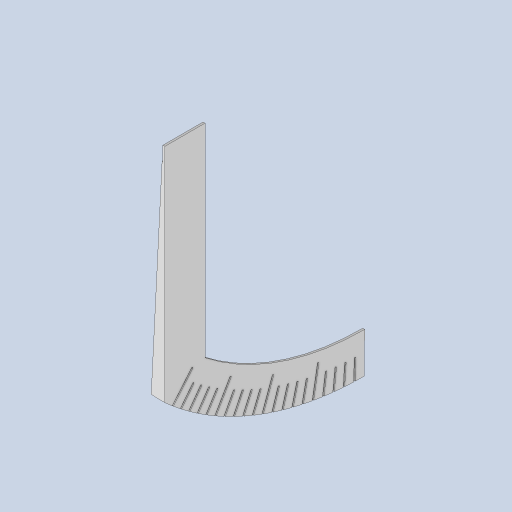
# Autodesk Inventor part: elev_angler
Saved by Autodesk Inventor 2024.1 (Build 281209000, 209)
## iProperties
Created: 2023-12-04
Part Number: elev_angler
Material: Generic
Document SubType Name: Modeling
Designer: dsdan
Density: 1 g/cm^3
Appearance: Default
Author: dsdan
Autodesk Inventor part; units mm, degrees
ref_plane "YZ Plane" through (0, 0, 0) normal (1, 0, 0) x (0, 1, 0)
ref_plane "XZ Plane" through (0, 0, 0) normal (0, 1, 0) x (-1, 0, 0)
ref_plane "XY Plane" through (0, 0, 0) normal (0, 0, 1) x (1, 0, 0)
sketch "Sketch1" plane through (0, 0, 0) normal (1, 0, 0) x (0, 1, 0)
  circle A0 centre (0, 0) radius 148.5
  line L0 (110.3263, 99.4) -> (-110.3263, 99.4)
  line L1 (0, 99.4) -> (0, 79.4)
  line L2 (0, 79.4) -> (-101.0341, 79.4)
  circle A1 centre (0, 0) radius 128.5
  line L3 (0, -148.5) -> (0, -128.5)
  point P0 (0, 99.4)
  dimension "d0" = 297
  dimension "d1" = 99.4
  dimension "d2" = 20
  dimension "d3" = 20
  dimension "d4" = 0
  constraints: 8 end point, 5 point on circle, 2 centre point, 2 midpoint, 2 vertical, 1 coincident, 1 horizontal, 1 perpendicular, 1 point on line
  measures "d0" diameter of A0
  measures "d1" distance from line of A0.centre L0
  measures "d2" radial gap between concentric circles of A0 A1
  measures "d3" distance between parallel lines of L0 L2
  measures "d4" distance from line of point (0, 99.4) L1
extrude "Extrusion1" add sketch "Sketch1" along normal mid plane 1 contours A0 L0 A1 L3 | L0 L1 L2 A1 picked at (-141.6144, 0.3829) picked at (-27.1455, 92.7333)
sketch "Sketch2" plane through (0.5, 0, 0) normal (1, 0, 0) x (0, 0, -1)
  line L0 (138.4156, -4.8336) -> (148.4095, -5.1826) construction
  line L1 (138.4287, -4.4588) -> (148.4226, -4.8078)
  line L2 (148.3965, -5.5573) -> (138.4025, -5.2084)
  arc A0 (138.4287, -4.4588) -> (138.4025, -5.2084) centre (138.4156, -4.8336) ccw
  arc A1 (148.3965, -5.5573) -> (148.4226, -4.8078) centre (148.4095, -5.1826) ccw
  arc A2 (-99.4, -110.3263) -> (148.5, 0) centre (0, 0) ccw projected
  line L3 (148.5, 0) -> (128.5, 0) projected
  line L4 (146.244, -25.7868) -> (131.4718, -23.182) construction
  line L5 (146.3091, -25.4175) -> (131.537, -22.8127)
  line L6 (131.4067, -23.5513) -> (146.1788, -26.1561)
  arc A3 (146.1788, -26.1561) -> (146.3091, -25.4175) centre (146.244, -25.7868) ccw
  arc A4 (131.537, -22.8127) -> (131.4067, -23.5513) centre (131.4718, -23.182) ccw
  point P0 (143.4126, -5.0081)
  point P1 (148.396, -5.5573)
  point P2 (148.4222, -4.8078)
  point P3 (138.8579, -24.4844)
  point P4 (146.1784, -26.156)
  point P5 (146.3086, -25.4174)
  dimension "d7" = 10
  dimension "d8" = 0.75
  dimension "d9" = 2
  dimension "d15" = 0.75
  dimension "d16" = 10
  dimension "d17" = 15
  constraints: 16 end point, 10 point on circle, 8 tangent, 4 centre point, 2 midpoint, 2 parallel, 2 point on line
  measures "d7" distance of L0.start L0.end
  measures "d8" distance between parallel lines of L2 L1
  measures "d9" angle of L3 L0
  measures "d15" diameter of A4
  measures "d16" angle of L3 L4
  measures "d17" distance of L4.start L4.end
extrude "Extrusion2" cut sketch "Sketch2" against normal blind 0.45 contours L1 A2 L2 A0
extrude "Extrusion3" cut sketch "Sketch2" against normal blind 0.45 contours L6 A4 L5 A2
pattern_circular "Circular Pattern1" count 65 over 128 about axis through (-10, 0, 0) along (-1, 0, 0) of "Extrusion2"
pattern_circular "Circular Pattern2" count 13 over 120 about axis through (-10, 0, 0) along (-1, 0, 0) of "Extrusion3"
sketch "Sketch3" plane through (-0.5, 0, 0) normal (-1, 0, 0) x (0, 0, 1)
  arc A0 (-148.5, 0) -> (99.4, -110.3263) centre (0, 0) ccw projected
  arc A1 (-146.7, 0) -> (112.3263, -94.3594) centre (0, 0) ccw
  line L0 (-148.5, 0) -> (-128.5, 0) projected
  line L1 (99.4, -110.3263) -> (99.4, 0) projected
  line L2 (-243.6606, 0) -> (171.6574, 0) projected
  point P0 (99.4, -107.8913)
  dimension "d23" = 1.8
  constraints: 2 point on circle, 1 centre point
  measures "d23" radial gap between concentric circles of A0 A1
revolve "Revolution1" add sketch "Sketch3" angle 3 about axis through (-0.5, 0, -10) along (0, 0, -1) contours L0 A1 L1 A0
sketch "Sketch4" plane through (0.5, -110.3263, 99.4) normal (0, 0, 1) x (1, 0, 0)
  circle A0 centre (-0.5, 110.3263) radius 2.95
  line L0 (-1, 0) -> (0, 0) projected
  line L1 (0, 110.3263) -> (0, 0) projected
  line L2 (-1, 110.3263) -> (0, 110.3263) projected
  line L3 (-1, 2.435) -> (-1, 110.3263) projected
  line L4 (0.075, -0.075) -> (-1, -0.075)
  arc A1 (-6.9581, 0.083) -> (-1, -0.075) centre (-1, 112.3372) ccw
  line L5 (-6.9581, 0.083) -> (-6.8239, 2.6445)
  arc A2 (-6.8239, 2.6445) -> (-1.075, 2.49) centre (-1, 112.3372) ccw
  line L6 (-1.075, 2.49) -> (-1.075, 110.2513)
  line L7 (-1.075, 110.2513) -> (0.075, 110.2513)
  line L8 (0.075, 110.2513) -> (0.075, -0.075)
  arc A3 (-6.6466, 2.5829) -> (-1, 2.435) centre (-1, 110.3263) ccw projected
  line L9 (-6.774, 0.1512) -> (-6.6466, 2.5829) projected
  arc A4 (-6.774, 0.1512) -> (-1, 0) centre (-1, 110.3263) ccw projected
  point P0 (0.075, 107.4329)
  point P1 (-1.075, 107.4329)
  dimension "d25" = 5.9
  dimension "d26" = 0.075
  constraints: 10 end point, 4 point on circle, 3 centre point, 1 midpoint, 2 other
  measures "d25" diameter of A0
  measures "d26" distance between parallel lines of L1 L8
extrude "Extrusion4" add sketch "Sketch4" along normal blind 5 and the other way blind 20 separate body contours A0 L8 L7 L1 L2 L3 L6 | L3 L2 L1 L7
split body "Split2" result two bodies by plane through (0, 0, 0) normal (0, 0, 1) bodies 1 first body at (0, -33.678, 86.0667)
ref_plane "Work Plane4" through (0, 0, -128.5) normal (0, 0, -1) x (-1, 0, 0)
sketch "Sketch6" plane through (0, 0, -128.5) normal (0, 0, 1) x (1, 0, 0)
  line L0 (0.05, -148.5) -> (-0.5, -148.5) projected
  line L1 (-0.5, 0) -> (-0.5, -148.5) projected
  line L2 (-0.5, 0) -> (0.5, 0) projected
  line L3 (0.5, -4.8078) -> (0.5, 0) projected
  line L4 (0.5, -4.8078) -> (0.05, -4.8078) projected
  line L5 (0.05, -4.8078) -> (0.05, -5.5573) projected
  line L6 (0.05, -5.5573) -> (0.5, -5.5573) projected
  line L7 (0.5, -9.9847) -> (0.5, -5.5573) projected
  line L8 (0.5, -9.9847) -> (0.05, -9.9847) projected
  line L9 (0.05, -9.9847) -> (0.05, -10.7329) projected
  line L10 (0.05, -10.7329) -> (0.5, -10.7329) projected
  line L11 (0.5, -15.1495) -> (0.5, -10.7329) projected
  line L12 (0.5, -15.1495) -> (0.05, -15.1495) projected
  line L13 (0.05, -15.1495) -> (0.05, -15.8954) projected
  line L14 (0.05, -15.8954) -> (0.5, -15.8954) projected
  line L15 (0.5, -20.2958) -> (0.5, -15.8954) projected
  line L16 (0.5, -20.2958) -> (0.05, -20.2958) projected
  line L17 (0.05, -20.2958) -> (0.05, -21.0385) projected
  line L18 (0.05, -21.0385) -> (0.5, -21.0385) projected
  line L19 (0.5, -25.4174) -> (0.5, -21.0385) projected
  line L20 (0.5, -25.4174) -> (0.05, -25.4174) projected
  line L21 (0.05, -25.4174) -> (0.05, -26.156) projected
  line L22 (0.05, -26.156) -> (0.5, -26.156) projected
  line L23 (0.5, -30.508) -> (0.5, -26.156) projected
  line L24 (0.5, -30.508) -> (0.05, -30.508) projected
  line L25 (0.05, -30.508) -> (0.05, -31.2416) projected
  line L26 (0.05, -31.2416) -> (0.5, -31.2416) projected
  line L27 (0.5, -35.5614) -> (0.5, -31.2416) projected
  line L28 (0.5, -35.5614) -> (0.05, -35.5614) projected
  line L29 (0.05, -35.5614) -> (0.05, -36.2891) projected
  line L30 (0.05, -36.2891) -> (0.5, -36.2891) projected
  line L31 (0.5, -40.5715) -> (0.5, -36.2891) projected
  line L32 (0.5, -40.5715) -> (0.05, -40.5715) projected
  line L33 (0.05, -40.5715) -> (0.05, -41.2925) projected
  line L34 (0.05, -41.2925) -> (0.5, -41.2925) projected
  line L35 (0.5, -45.5322) -> (0.5, -41.2925) projected
  line L36 (0.5, -45.5322) -> (0.05, -45.5322) projected
  line L37 (0.05, -45.5322) -> (0.05, -46.2455) projected
  line L38 (0.05, -46.2455) -> (0.5, -46.2455) projected
  line L39 (0.5, -50.4374) -> (0.5, -46.2455) projected
  line L40 (0.5, -50.4374) -> (0.05, -50.4374) projected
  line L41 (0.05, -50.4374) -> (0.05, -51.1422) projected
  line L42 (0.05, -51.1422) -> (0.5, -51.1422) projected
  line L43 (0.5, -55.2812) -> (0.5, -51.1422) projected
  line L44 (0.5, -55.2812) -> (0.05, -55.2812) projected
  line L45 (0.05, -55.2812) -> (0.05, -55.9766) projected
  line L46 (0.05, -55.9766) -> (0.5, -55.9766) projected
  line L47 (0.5, -60.0576) -> (0.5, -55.9766) projected
  line L48 (0.5, -60.0576) -> (0.05, -60.0576) projected
  line L49 (0.05, -60.0576) -> (0.05, -60.7428) projected
  line L50 (0.05, -60.7428) -> (0.5, -60.7428) projected
  line L51 (0.5, -64.7609) -> (0.5, -60.7428) projected
  line L52 (0.5, -64.7609) -> (0.05, -64.7609) projected
  line L53 (0.05, -64.7609) -> (0.05, -65.435) projected
  line L54 (0.05, -65.435) -> (0.5, -65.435) projected
  line L55 (0.5, -69.3852) -> (0.5, -65.435) projected
  line L56 (0.5, -69.3852) -> (0.05, -69.3852) projected
  line L57 (0.05, -69.3852) -> (0.05, -70.0474) projected
  line L58 (0.05, -70.0474) -> (0.5, -70.0474) projected
  line L59 (0.5, -73.925) -> (0.5, -70.0474) projected
  line L60 (0.5, -73.925) -> (0.05, -73.925) projected
  line L61 (0.05, -73.925) -> (0.05, -74.5745) projected
  line L62 (0.05, -74.5745) -> (0.5, -74.5745) projected
  line L63 (0.5, -78.3747) -> (0.5, -74.5745) projected
  line L64 (0.5, -78.3747) -> (0.05, -78.3747) projected
  line L65 (0.05, -78.3747) -> (0.05, -79.0108) projected
  line L66 (0.05, -79.0108) -> (0.5, -79.0108) projected
  line L67 (0.5, -82.729) -> (0.5, -79.0108) projected
  line L68 (0.5, -82.729) -> (0.05, -82.729) projected
  line L69 (0.05, -82.729) -> (0.05, -83.3508) projected
  line L70 (0.05, -83.3508) -> (0.5, -83.3508) projected
  line L71 (0.5, -86.9825) -> (0.5, -83.3508) projected
  line L72 (0.5, -86.9825) -> (0.05, -86.9825) projected
  line L73 (0.05, -86.9825) -> (0.05, -87.5892) projected
  line L74 (0.05, -87.5892) -> (0.5, -87.5892) projected
  line L75 (0.5, -91.1299) -> (0.5, -87.5892) projected
  line L76 (0.5, -91.1299) -> (0.05, -91.1299) projected
  line L77 (0.05, -91.1299) -> (0.05, -91.7209) projected
  line L78 (0.05, -91.7209) -> (0.5, -91.7209) projected
  line L79 (0.5, -95.1664) -> (0.5, -91.7209) projected
  line L80 (0.5, -95.1664) -> (0.05, -95.1664) projected
  line L81 (0.05, -95.1664) -> (0.05, -95.7409) projected
  line L82 (0.05, -95.7409) -> (0.5, -95.7409) projected
  line L83 (0.5, -99.0869) -> (0.5, -95.7409) projected
  line L84 (0.5, -99.0869) -> (0.05, -99.0869) projected
  line L85 (0.05, -99.0869) -> (0.05, -99.6443) projected
  line L86 (0.05, -99.6443) -> (0.5, -99.6443) projected
  line L87 (0.5, -102.8867) -> (0.5, -99.6443) projected
  line L88 (0.5, -102.8867) -> (0.05, -102.8867) projected
  line L89 (0.05, -102.8867) -> (0.05, -103.4262) projected
  line L90 (0.05, -103.4262) -> (0.5, -103.4262) projected
  line L91 (0.5, -106.5611) -> (0.5, -103.4262) projected
  line L92 (0.5, -106.5611) -> (0.05, -106.5611) projected
  line L93 (0.05, -106.5611) -> (0.05, -107.0821) projected
  line L94 (0.05, -107.0821) -> (0.5, -107.0821) projected
  line L95 (0.5, -110.1057) -> (0.5, -107.0821) projected
  line L96 (0.5, -110.1057) -> (0.05, -110.1057) projected
  line L97 (0.05, -110.1057) -> (0.05, -110.6076) projected
  line L98 (0.05, -110.6076) -> (0.5, -110.6076) projected
  line L99 (0.5, -113.5162) -> (0.5, -110.6076) projected
  line L100 (0.5, -113.5162) -> (0.05, -113.5162) projected
  line L101 (0.05, -113.5162) -> (0.05, -113.9983) projected
  line L102 (0.05, -113.9983) -> (0.5, -113.9983) projected
  line L103 (0.5, -116.7884) -> (0.5, -113.9983) projected
  line L104 (0.5, -116.7884) -> (0.05, -116.7884) projected
  line L105 (0.05, -116.7884) -> (0.05, -117.2501) projected
  line L106 (0.05, -117.2501) -> (0.5, -117.2501) projected
  line L107 (0.5, -119.9182) -> (0.5, -117.2501) projected
  line L108 (0.5, -119.9182) -> (0.05, -119.9182) projected
  line L109 (0.05, -119.9182) -> (0.05, -120.3591) projected
  line L110 (0.05, -120.3591) -> (0.5, -120.3591) projected
  line L111 (0.5, -122.902) -> (0.5, -120.3591) projected
  line L112 (0.5, -122.902) -> (0.05, -122.902) projected
  line L113 (0.05, -122.902) -> (0.05, -123.3214) projected
  line L114 (0.05, -123.3214) -> (0.5, -123.3214) projected
  line L115 (0.5, -125.736) -> (0.5, -123.3214) projected
  line L116 (0.5, -125.736) -> (0.05, -125.736) projected
  line L117 (0.05, -125.736) -> (0.05, -126.1335) projected
  line L118 (0.05, -126.1335) -> (0.5, -126.1335) projected
  line L119 (0.5, -128.4169) -> (0.5, -126.1335) projected
  line L120 (0.5, -128.4169) -> (0.05, -128.4169) projected
  line L121 (0.05, -128.4169) -> (0.05, -128.7919) projected
  line L122 (0.05, -128.7919) -> (0.5, -128.7919) projected
  line L123 (0.5, -130.9412) -> (0.5, -128.7919) projected
  line L124 (0.5, -130.9412) -> (0.05, -130.9412) projected
  line L125 (0.05, -130.9412) -> (0.05, -131.2934) projected
  line L126 (0.05, -131.2934) -> (0.5, -131.2934) projected
  line L127 (0.5, -133.3061) -> (0.5, -131.2934) projected
  line L128 (0.5, -133.3061) -> (0.05, -133.3061) projected
  line L129 (0.05, -133.3061) -> (0.05, -133.6349) projected
  line L130 (0.05, -133.6349) -> (0.5, -133.6349) projected
  line L131 (0.5, -135.5085) -> (0.5, -133.6349) projected
  line L132 (0.5, -135.5085) -> (0.05, -135.5085) projected
  line L133 (0.05, -135.5085) -> (0.05, -135.8136) projected
  line L134 (0.05, -135.8136) -> (0.5, -135.8136) projected
  line L135 (0.5, -137.5459) -> (0.5, -135.8136) projected
  line L136 (0.5, -137.5459) -> (0.05, -137.5459) projected
  line L137 (0.05, -137.5459) -> (0.05, -137.8268) projected
  line L138 (0.05, -137.8268) -> (0.5, -137.8268) projected
  line L139 (0.5, -139.4157) -> (0.5, -137.8268) projected
  line L140 (0.5, -139.4157) -> (0.05, -139.4157) projected
  line L141 (0.05, -139.4157) -> (0.05, -139.6722) projected
  line L142 (0.05, -139.6722) -> (0.5, -139.6722) projected
  line L143 (0.5, -141.1156) -> (0.5, -139.6722) projected
  line L144 (0.5, -141.1156) -> (0.05, -141.1156) projected
  line L145 (0.05, -141.1156) -> (0.05, -141.3473) projected
  line L146 (0.05, -141.3473) -> (0.5, -141.3473) projected
  line L147 (0.5, -142.6435) -> (0.5, -141.3473) projected
  line L148 (0.5, -142.6435) -> (0.05, -142.6435) projected
  line L149 (0.05, -142.6435) -> (0.05, -142.8503) projected
  line L150 (0.05, -142.8503) -> (0.5, -142.8503) projected
  line L151 (0.5, -143.9977) -> (0.5, -142.8503) projected
  line L152 (0.5, -143.9977) -> (0.05, -143.9977) projected
  line L153 (0.05, -143.9977) -> (0.05, -144.1792) projected
  line L154 (0.05, -144.1792) -> (0.5, -144.1792) projected
  line L155 (0.5, -145.1765) -> (0.5, -144.1792) projected
  line L156 (0.5, -145.1765) -> (0.05, -145.1765) projected
  line L157 (0.05, -145.1765) -> (0.05, -145.3324) projected
  line L158 (0.05, -145.3324) -> (0.5, -145.3324) projected
  line L159 (0.5, -146.1784) -> (0.5, -145.3324) projected
  line L160 (0.5, -146.1784) -> (0.05, -146.1784) projected
  line L161 (0.05, -146.1784) -> (0.05, -146.3086) projected
  line L162 (0.05, -146.3086) -> (0.5, -146.3086) projected
  line L163 (0.5, -147.0021) -> (0.5, -146.3086) projected
  line L164 (0.5, -147.0021) -> (0.05, -147.0021) projected
  line L165 (0.05, -147.0021) -> (0.05, -147.1065) projected
  line L166 (0.05, -147.1065) -> (0.5, -147.1065) projected
  line L167 (0.5, -147.6468) -> (0.5, -147.1065) projected
  line L168 (0.5, -147.6468) -> (0.05, -147.6468) projected
  line L169 (0.05, -147.6468) -> (0.05, -147.7252) projected
  line L170 (0.05, -147.7252) -> (0.5, -147.7252) projected
  line L171 (0.5, -148.1116) -> (0.5, -147.7252) projected
  line L172 (0.5, -148.1116) -> (0.05, -148.1116) projected
  line L173 (0.05, -148.1116) -> (0.05, -148.1639) projected
  line L174 (0.05, -148.1639) -> (0.5, -148.1639) projected
  line L175 (0.5, -148.396) -> (0.5, -148.1639) projected
  line L176 (0.5, -148.396) -> (0.05, -148.396) projected
  line L177 (0.05, -148.396) -> (0.05, -148.4222) projected
  line L178 (0.05, -148.4222) -> (0.5, -148.4222) projected
  line L179 (0.5, -148.4995) -> (0.5, -148.4222) projected
  line L180 (0.5, -148.4995) -> (0.05, -148.4995) projected
  line L181 (0.05, -148.4995) -> (0.05, -148.5) projected
  circle A0 centre (0, 0) radius 3.5
  circle A1 centre (0, 0) radius 0.6
  line L182 (0, 0) -> (0, 0.5)
  line L183 (0, 0.5) -> (3.4641, 0.5)
  line L184 (0, 0.5) -> (-3.4641, 0.5)
  point P0 (0, 0.25)
  point P1 (-0.3317, 0.5)
  point P2 (0.3317, 0.5)
  dimension "d33" = 7
  dimension "d34" = 1.2
  dimension "d35" = 0.5
  dimension "d36" = 1
  constraints: 6 end point, 2 centre point, 2 coincident, 2 horizontal, 2 point on circle, 1 midpoint, 1 vertical
  measures "d33" diameter of A0
  measures "d34" diameter of A1
  measures "d35" distance of L182.start L182.end
  measures "d36" distance of L1.start L2.end
extrude "Extrusion5" add sketch "Sketch6" against normal blind 15 separate body contours A0 L183 A1 L184
sketch "Sketch7" plane through (0, 0, -143.5) normal (0, 0, -1) x (-1, 0, 0)
  arc A0 (3.4641, 0.5) -> (-3.4641, 0.5) centre (0, 0) ccw projected
  line L0 (-3.4641, 0.5) -> (3.4641, 0.5)
  line L1 (3.4641, 0.5) -> (3.4641, 6)
  line L2 (3.4641, 6) -> (-3.4641, 6)
  line L3 (-3.4641, 6) -> (-3.4641, 0.5)
  arc A1 (0.3317, 0.5) -> (-0.3317, 0.5) centre (0, 0) ccw projected
  line L4 (-4.5714, 3.05) -> (7.081, 3.05)
  line L5 (0.5, 0) -> (-0.5, 0) projected
  point P0 (0, 0)
  point P1 (-3.4641, 3.05)
  point P2 (3.4641, 3.05)
  dimension "d40" = 5.5
  dimension "d41" = 3.05
  constraints: 10 end point, 2 horizontal, 2 parallel, 1 perpendicular, 1 point on line
  measures "d40" distance between parallel lines of L0 L2
  measures "d41" distance between parallel lines of L5 L4
extrude "Extrusion6" add sketch "Sketch7" along normal blind 20 contours L4 A0 | A0 L4 L3 L2 L1 bodies 5
extrude "Extrusion7" add sketch "Sketch7" against normal up to surface (15 mm away) contours A0 L4 L1 | A0 L4 L3 L2 L1 | A0 L3 L4 bodies 5
sketch "Sketch8" plane through (-3.4641, 6, -143.5) normal (0, 1, 0) x (1, 0, 0)
  line L0 (3.4641, 16.0677) -> (3.4641, 9.0677) construction
  line L1 (1.4141, 16.0677) -> (1.4141, 9.0677)
  line L2 (5.5141, 9.0677) -> (5.5141, 16.0677)
  arc A0 (5.5141, 16.0677) -> (1.4141, 16.0677) centre (3.4641, 16.0677) ccw
  arc A1 (1.4141, 9.0677) -> (5.5141, 9.0677) centre (3.4641, 9.0677) ccw
  line L3 (0, 20) -> (6.9282, 20) projected
  point P0 (3.4641, -143.5)
  point P1 (3.4641, 12.5677)
  point P2 (3.4641, 20)
  point P3 (3.4641, 20)
  dimension "d46" = 4.1
  dimension "d47" = 7
  constraints: 8 end point, 4 point on circle, 4 tangent, 3 midpoint, 2 centre point, 1 parallel, 1 point on line, 1 vertical
  measures "d46" diameter of A1
  measures "d47" distance of L0.start L0.end
extrude "Extrusion8" cut sketch "Sketch8" against normal through all bodies 5
sketch "Sketch10" plane through (0.5, -110.3263, 99.4) normal (0, 0, 1) x (1, 0, 0)
  line L0 (-1, 2.435) -> (-1, 110.3263) projected
  line L1 (-1, 103.2662) -> (-1.37, 103.2662)
  arc A0 (-6.6466, 2.5829) -> (-1, 2.435) centre (-1, 110.3263) ccw projected
  line L2 (-1.37, 103.2662) -> (-6.6466, 2.5829)
  line L3 (-6.774, 0.1512) -> (-6.6466, 2.5829) projected
  line L4 (-6.7592, 0.435) -> (-1, 0.435)
  line L5 (-1, 0.435) -> (-1, 2.435)
  point P0 (-0.5, 110.3263)
  dimension "d52" = 2
  constraints: 8 end point, 2 horizontal, 2 point on line, 1 collinear, 1 perpendicular
  measures "d52" distance from line of L0.start L4
extrude "Extrusion9" add sketch "Sketch10" against normal blind 1.8 bodies 3
equation "\"d35\" = 0.5 * d36"
body "Solid2"
body "Solid7"
body "Solid5"
body "Solid6"
